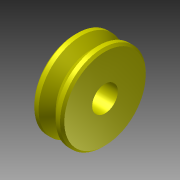
# Autodesk Inventor part: 13_0204_050
Saved by Autodesk Inventor 2012 SP1 (Build 160190100, 190)
## iProperties
Created: 2013-04-08
Part Number: 13_0204_050
Material: Default
Document SubType Name: Modeling
Designer: vogel
Density: 1 g/cm^3
Author: vogel
Autodesk Inventor part; units mm, degrees
ref_plane "YZ Plane" through (0, 0, 0) normal (1, 0, 0) x (0, 1, 0)
ref_plane "XZ Plane" through (0, 0, 0) normal (0, 1, 0) x (-1, 0, 0)
ref_plane "XY Plane" through (0, 0, 0) normal (0, 0, 1) x (1, 0, 0)
sketch "Skizze1" plane through (0, 0, 0) normal (0, 0, 1) x (1, 0, 0)
  line L0 (-4.9, 0) -> (4.9, 0) projected
  line L1 (0, -2) -> (0, 12) projected
  line L2 (3.5, 10) -> (3.5, 3)
  line L3 (3.5, 3) -> (-3.5, 3)
  line L4 (-3.5, 3) -> (-3.5, 10)
  line L5 (-2, 10) -> (0, 8)
  line L6 (0, 8) -> (2, 10)
  line L7 (-3.5, 10) -> (-2, 10)
  line L8 (2, 10) -> (3.5, 10)
  circle A0 centre (0, 8.3536) radius 0.25
  point P0 (0, 0)
  dimension "d0" = 6
  dimension "d1" = 20
  dimension "d2" = 7
  dimension "d3" = 90
  dimension "d4" = 16
  dimension "d9" = 0.5
  dimension "d10" = 16.7071
  constraints: 14 end point, 3 parallel, 2 horizontal, 2 perpendicular, 2 point on line, 1 centre point, 1 collinear, 1 tangent, 2 other
  measures "d0" diameter of L3 L0
  measures "d1" diameter of L7 L0
  measures "d2" distance of L2.end L3.end
  measures "d3" angle of L6 L5
  measures "d4" diameter of L5.end L0
  measures "d9" diameter of A0
  measures "d10" diameter of A0.centre L0
revolve "Umdrehung1" add sketch "Skizze1" angle 360 about axis through (-10, 0, 0) along (1, 0, 0) contours L3 L4 L7 L5 L1 | L1 L6 L8 L2 L3
chamfer "Fase1" distance 0.5 angle 45 2 edges at (-3.5, -10, 0) (3.5, -10, 0)
